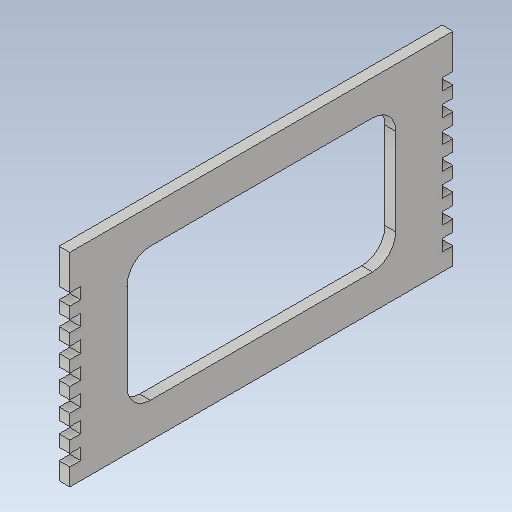
# Autodesk Inventor part: open_case
Saved by Autodesk Inventor 2020 (Build 240168000, 168)
## iProperties
Created: 2019-12-18
Part Number: open_case
Material: Generic
Document SubType Name: Modeling
Designer: fabfarm
Density: 1 g/cm^3
Appearance: Default
Author: fabfarm
Autodesk Inventor part; units mm, degrees
ref_plane "YZ Plane" through (0, 0, 0) normal (1, 0, 0) x (0, 1, 0)
ref_plane "XZ Plane" through (0, 0, 0) normal (0, 1, 0) x (-1, 0, 0)
ref_plane "XY Plane" through (0, 0, 0) normal (0, 0, 1) x (1, 0, 0)
sketch "Sketch1" plane through (0, 0, 0) normal (1, 0, 0) x (0, 1, 0)
  line L0 (-175, -330) -> (175, -330)
  line L1 (175, -330) -> (175, 330)
  line L2 (175, 330) -> (-175, 330)
  line L3 (-175, 330) -> (-175, -330)
  line L4 (-175, -330) -> (175, 330) construction
  line L5 (175, -330) -> (-175, 330) construction
  point P0 (0, 0)
  dimension "d0" = 660
  dimension "d1" = 350
  constraints: 12 end point, 2 midpoint, 2 parallel, 1 horizontal, 1 perpendicular
  measures "d0" distance of L0.end L1.end
  measures "d1" distance of L0.start L0.end
extrude "Extrusion1" add sketch "Sketch1" along normal blind 18.55
sketch "Sketch2" plane through (18.55, 0, 0) normal (1, 0, 0) x (0, 0, -1)
  line L0 (-330, 175) -> (-330, -175) projected
  line L1 (-330, 95) -> (-311.45, 95)
  line L2 (-311.45, 95) -> (-311.45, 115)
  line L3 (-311.45, 115) -> (-330, 115)
  line L4 (-330, 115) -> (-330, 95)
  line L5 (330, 175) -> (-330, 175) projected
  line L6 (-330, 55) -> (-311.45, 55)
  line L7 (-311.45, 55) -> (-311.45, 75)
  line L8 (-311.45, 75) -> (-330, 75)
  line L9 (-330, 75) -> (-330, 55)
  line L10 (-330, 15) -> (-311.45, 15)
  line L11 (-311.45, 15) -> (-311.45, 35)
  line L12 (-311.45, 35) -> (-330, 35)
  line L13 (-330, 35) -> (-330, 15)
  line L14 (-330, -25) -> (-311.45, -25)
  line L15 (-311.45, -25) -> (-311.45, -5)
  line L16 (-311.45, -5) -> (-330, -5)
  line L17 (-330, -5) -> (-330, -25)
  line L18 (-330, -65) -> (-311.45, -65)
  line L19 (-311.45, -65) -> (-311.45, -45)
  line L20 (-311.45, -45) -> (-330, -45)
  line L21 (-330, -45) -> (-330, -65)
  line L22 (-330, -105) -> (-311.45, -105)
  line L23 (-311.45, -105) -> (-311.45, -85)
  line L24 (-311.45, -85) -> (-330, -85)
  line L25 (-330, -85) -> (-330, -105)
  line L26 (-330, -145) -> (-311.45, -145)
  line L27 (-311.45, -145) -> (-311.45, -125)
  line L28 (-311.45, -125) -> (-330, -125)
  line L29 (-330, -125) -> (-330, -145)
  point P0 (0, 0)
  dimension "d4" = 80
  dimension "d5" = 18.55
  dimension "d6" = 20
  dimension "d9" = 40
  constraints: 56 end point, 2 parallel, 1 horizontal, 1 perpendicular, 1 point on line, 1 vertical, 48 other
  measures "d4" distance between parallel lines of L5 L1
  measures "d5" distance of L2.end L3.end
  measures "d6" distance of L1.end L2.end
  measures "d9" distance of L1.start L6.start
extrude "Extrusion2" cut sketch "Sketch2" against normal blind 18.55
mirror "Mirror1" about plane through (0, 0, 0) normal (0, 0, 1) of "Extrusion2"
sketch "Sketch3" plane through (18.55, 0, 0) normal (1, 0, 0) x (0, 0, -1)
  line L0 (191.45, -115) -> (-191.45, -115)
  line L1 (-231.45, -75) -> (-231.45, 75)
  line L2 (-191.45, 115) -> (191.45, 115)
  line L3 (231.45, 75) -> (231.45, -75)
  line L4 (231.45, -115) -> (-231.45, 115) construction
  line L5 (-231.45, -115) -> (231.45, 115) construction
  line L6 (-330, 115) -> (-311.45, 115) projected
  line L7 (-311.45, -125) -> (-311.45, -145) projected
  arc A0 (-191.45, 115) -> (-231.45, 75) centre (-191.45, 75) ccw
  arc A1 (-231.45, -75) -> (-191.45, -115) centre (-191.45, -75) ccw
  arc A2 (231.45, 75) -> (191.45, 115) centre (191.45, 75) ccw
  arc A3 (191.45, -115) -> (231.45, -75) centre (191.45, -75) ccw
  point P0 (0, 0)
  dimension "d16" = 80
  dimension "d17" = 40
  constraints: 12 end point, 8 point on circle, 8 point on line, 8 tangent, 4 centre point, 3 equal radius, 2 midpoint, 2 parallel, 1 collinear, 1 horizontal, 1 perpendicular
  measures "d16" distance between parallel lines of L7 L1
  measures "d17" radius of A0
extrude "Extrusion3" cut sketch "Sketch3" against normal blind 18.55
body "Solid1"
